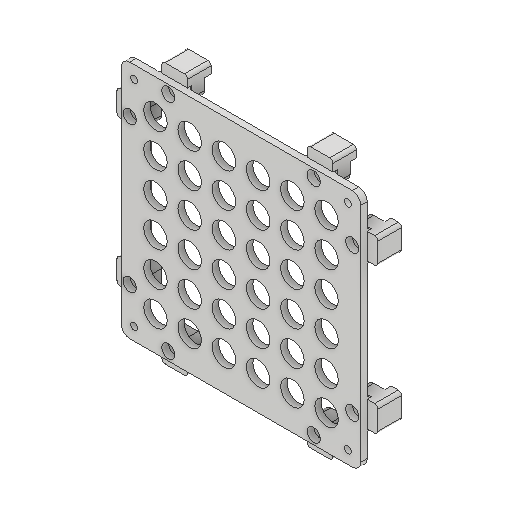
# Autodesk Inventor part: 3DP_PLA_Test_Tube_Plate
Saved by Autodesk Inventor 2025 (Build 290162010, 162A)
## iProperties
Created: 2018-06-16
Part Number: 3DP_PLA_Test_Tube_Plate
Material: ABS Plastic
Document SubType Name: Modeling
Designer: Andrzej
Density: 1.06 g/cm^3
Appearance: Smooth - White
Author: Andrzej
Autodesk Inventor part; units mm, degrees
ref_plane "YZ Plane" through (0, 0, 0) normal (1, 0, 0) x (0, 1, 0)
ref_plane "XZ Plane" through (0, 0, 0) normal (0, 1, 0) x (-1, 0, 0)
ref_plane "XY Plane" through (0, 0, 0) normal (0, 0, 1) x (1, 0, 0)
sketch "Sketch1" plane through (0, 0, 0) normal (0, 0, 1) x (1, 0, 0)
  line L0 (-56, 56) -> (56, 56)
  line L1 (56, 56) -> (56, -56)
  line L2 (56, -56) -> (-56, -56)
  line L3 (-56, -56) -> (-56, 56)
  circle A0 centre (-40, 40) radius 5.5
  circle A1 centre (-24, 40) radius 5.5
  circle A2 centre (-8, 40) radius 5.5
  circle A3 centre (8, 40) radius 5.5
  circle A4 centre (24, 40) radius 5.5
  circle A5 centre (40, 40) radius 5.5
  circle A6 centre (-40, 24) radius 5.5
  circle A7 centre (-24, 24) radius 5.5
  circle A8 centre (-8, 24) radius 5.5
  circle A9 centre (8, 24) radius 5.5
  circle A10 centre (24, 24) radius 5.5
  circle A11 centre (40, 24) radius 5.5
  circle A12 centre (-40, 8) radius 5.5
  circle A13 centre (-24, 8) radius 5.5
  circle A14 centre (-8, 8) radius 5.5
  circle A15 centre (8, 8) radius 5.5
  circle A16 centre (24, 8) radius 5.5
  circle A17 centre (40, 8) radius 5.5
  circle A18 centre (-40, -8) radius 5.5
  circle A19 centre (-24, -8) radius 5.5
  circle A20 centre (-8, -8) radius 5.5
  circle A21 centre (8, -8) radius 5.5
  circle A22 centre (24, -8) radius 5.5
  circle A23 centre (40, -8) radius 5.5
  circle A24 centre (-40, -24) radius 5.5
  circle A25 centre (-24, -24) radius 5.5
  circle A26 centre (-8, -24) radius 5.5
  circle A27 centre (8, -24) radius 5.5
  circle A28 centre (24, -24) radius 5.5
  circle A29 centre (40, -24) radius 5.5
  circle A30 centre (-40, -40) radius 5.5
  circle A31 centre (-24, -40) radius 5.5
  circle A32 centre (-8, -40) radius 5.5
  circle A33 centre (8, -40) radius 5.5
  circle A34 centre (24, -40) radius 5.5
  circle A35 centre (40, -40) radius 5.5
  point P0 (0, 0)
  point P1 (-50, 50)
  point P2 (50, 50)
  point P3 (-50, -50)
  point P4 (50, -50)
  dimension "d0" = 112
  dimension "d1" = 112
  dimension "d2" = 11
  dimension "d3" = 16
  dimension "d4" = 16
  dimension "d7" = 16
  dimension "d10" = 16
  dimension "d19" = 6
  dimension "d20" = 6
  dimension "d23" = 6
  dimension "d25" = 6
  dimension "d34" = 56
  dimension "d35" = 56
  constraints: 36 centre point, 8 end point, 2 horizontal, 2 horizontal alignment, 2 parallel, 2 vertical alignment, 1 perpendicular, 1 vertical, 70 other
  measures "d0" distance of L1.end L2.end
  measures "d1" distance of L0.end L1.end
  measures "d2" diameter of A0
  measures "d3" distance from line of L3 A0.centre
  measures "d4" distance from line of L0 A0.centre
  measures "d7" distance of A0.centre A1.centre
  measures "d10" distance of A0.centre A6.centre
  measures "d19" distance from line of L3 point (-50, 50)
  measures "d20" distance from line of L0 point (-50, 50)
  measures "d23" distance from line of L2 point (-50, -50)
  measures "d25" distance from line of L1 point (50, 50)
  measures "d34" distance from line of point (0, 0) L2
  measures "d35" distance from line of point (0, 0) L3
extrude "Extrusion2" add sketch "Sketch1" along normal blind 3
hole "Hole1" at (50, 50, 0) at (-50, -50, 0) at (-50, 50, 0) at (50, -50, 0) direction (0, 0, 1) diameter 3.25 end through all
fillet "Fillet1" radius 4 4 edges at (56, 56, 1.5) (56, -56, 1.5) (-56, -56, 1.5) (-56, 56, 1.5)
sketch "Sketch3" plane through (0, 0, 0) normal (0, 0, -1) x (-1, 0, 0)
  arc A0 (56, 52) -> (52, 56) centre (52, 52) ccw projected
  line L0 (52, 56) -> (-52, 56) projected
  arc A1 (-52, 56) -> (-56, 52) centre (-52, 52) ccw projected
  line L1 (-56, 52) -> (-56, -52) projected
  arc A2 (-56, -52) -> (-52, -56) centre (-52, -52) ccw projected
  line L2 (-52, -56) -> (52, -56) projected
  arc A3 (52, -56) -> (56, -52) centre (52, -52) ccw projected
  line L3 (56, -52) -> (56, 52) projected
  circle A4 centre (50, 50) radius 1.625 projected
  circle A5 centre (-50, 50) radius 1.625 projected
  circle A6 centre (50, -50) radius 1.625 projected
  circle A7 centre (-40, -40) radius 5.5 projected
  circle A8 centre (-24, -40) radius 5.5 projected
  circle A9 centre (-8, -40) radius 5.5 projected
  circle A10 centre (8, -40) radius 5.5 projected
  circle A11 centre (24, -40) radius 5.5 projected
  circle A12 centre (40, -40) radius 5.5 projected
  circle A13 centre (-40, -24) radius 5.5 projected
  circle A14 centre (-24, -24) radius 5.5 projected
  circle A15 centre (-8, -24) radius 5.5 projected
  circle A16 centre (8, -24) radius 5.5 projected
  circle A17 centre (24, -24) radius 5.5 projected
  circle A18 centre (40, -24) radius 5.5 projected
  circle A19 centre (-40, -8) radius 5.5 projected
  circle A20 centre (-24, -8) radius 5.5 projected
  circle A21 centre (-8, -8) radius 5.5 projected
  circle A22 centre (8, -8) radius 5.5 projected
  circle A23 centre (24, -8) radius 5.5 projected
  circle A24 centre (40, -8) radius 5.5 projected
  circle A25 centre (-40, 8) radius 5.5 projected
  circle A26 centre (-24, 8) radius 5.5 projected
  circle A27 centre (-8, 8) radius 5.5 projected
  circle A28 centre (8, 8) radius 5.5 projected
  circle A29 centre (24, 8) radius 5.5 projected
  circle A30 centre (40, 8) radius 5.5 projected
  circle A31 centre (-40, 24) radius 5.5 projected
  circle A32 centre (-24, 24) radius 5.5 projected
  circle A33 centre (-8, 24) radius 5.5 projected
  circle A34 centre (8, 24) radius 5.5 projected
  circle A35 centre (24, 24) radius 5.5 projected
  circle A36 centre (40, 24) radius 5.5 projected
  circle A37 centre (-40, 40) radius 5.5 projected
  circle A38 centre (-24, 40) radius 5.5 projected
  circle A39 centre (-8, 40) radius 5.5 projected
  circle A40 centre (8, 40) radius 5.5 projected
  circle A41 centre (24, 40) radius 5.5 projected
  circle A42 centre (40, 40) radius 5.5 projected
  circle A43 centre (-50, -50) radius 1.625 projected
  line L4 (-52, -56) -> (52, -56) projected
  line L5 (40, -56) -> (28, -56)
  line L6 (28, -56) -> (28, -61)
  line L7 (28, -61) -> (40, -61)
  line L8 (40, -61) -> (40, -56)
  line L9 (40, -56) -> (28, -56)
  line L10 (28, -56) -> (28, -48)
  line L11 (28, -48) -> (40, -48)
  line L12 (40, -48) -> (40, -56)
  line L13 (0, 62.6646) -> (0, -67.1052)
  line L14 (75.0583, 0) -> (-85.8021, 0)
  line L15 (-40, -56) -> (-28, -56)
  line L16 (-28, -56) -> (-28, -61)
  line L17 (-28, -61) -> (-40, -61)
  line L18 (-40, -61) -> (-40, -56)
  line L19 (-40, -56) -> (-28, -56)
  line L20 (-28, -56) -> (-28, -48)
  line L21 (-28, -48) -> (-40, -48)
  line L22 (-40, -48) -> (-40, -56)
  line L23 (40, 56) -> (28, 56)
  line L24 (28, 56) -> (28, 61)
  line L25 (28, 61) -> (40, 61)
  line L26 (40, 61) -> (40, 56)
  line L27 (40, 56) -> (28, 56)
  line L28 (28, 56) -> (28, 48)
  line L29 (28, 48) -> (40, 48)
  line L30 (40, 48) -> (40, 56)
  line L31 (-28, 56) -> (-28, 48)
  line L32 (-28, 48) -> (-40, 48)
  line L33 (-40, 48) -> (-40, 56)
  line L34 (-40, 56) -> (-28, 56)
  line L35 (-40, 56) -> (-28, 56)
  line L36 (-28, 61) -> (-40, 61)
  line L37 (-40, 61) -> (-40, 56)
  line L38 (-28, 56) -> (-28, 61)
  line L39 (-48, -28) -> (-48, -40)
  line L40 (-48, -40) -> (-56, -40)
  line L41 (-56, -28) -> (-48, -28)
  line L42 (-56, -40) -> (-56, -28)
  line L43 (-56, -40) -> (-56, -28)
  line L44 (-61, -40) -> (-56, -40)
  line L45 (-61, -28) -> (-61, -40)
  line L46 (-56, -28) -> (-61, -28)
  line L47 (-48, 28) -> (-48, 40)
  line L48 (-56, 28) -> (-48, 28)
  line L49 (-48, 40) -> (-56, 40)
  line L50 (-56, 40) -> (-56, 28)
  line L51 (-56, 40) -> (-56, 28)
  line L52 (-56, 28) -> (-61, 28)
  line L53 (-61, 28) -> (-61, 40)
  line L54 (-61, 40) -> (-56, 40)
  line L55 (56, -28) -> (48, -28)
  line L56 (48, -28) -> (48, -40)
  line L57 (56, -28) -> (61, -28)
  line L58 (48, -40) -> (56, -40)
  line L59 (56, -40) -> (56, -28)
  line L60 (56, -40) -> (56, -28)
  line L61 (61, -28) -> (61, -40)
  line L62 (61, -40) -> (56, -40)
  line L63 (48, 40) -> (56, 40)
  line L64 (61, 28) -> (61, 40)
  line L65 (56, 28) -> (61, 28)
  line L66 (61, 40) -> (56, 40)
  line L67 (48, 28) -> (48, 40)
  line L68 (56, 28) -> (48, 28)
  line L69 (56, 40) -> (56, 28)
  line L70 (56, 40) -> (56, 28)
  point P0 (0, 0)
  point P1 (56, 28)
  point P2 (-28, 56)
  point P3 (-56, 28)
  point P4 (-56, -28)
  point P5 (-28, -56)
  point P6 (56, 28)
  point P7 (-28, 56)
  point P8 (-56, 28)
  point P9 (-56, -28)
  point P10 (-28, -56)
  dimension "d36" = 12
  dimension "d37" = 5
  dimension "d38" = 8
  dimension "d39" = 16
  dimension "d42" = 270
  constraints: 132 end point, 21 symmetric about line, 11 point on line, 4 parallel, 3 horizontal, 2 perpendicular, 1 vertical, 61 other
  measures "d36" distance of L7.end L6.end
  measures "d37" distance of L6.end L5.end
  measures "d38" distance of L9.end L10.end
  measures "d39" distance between parallel lines of L3 L8
extrude "Extrusion3" add sketch "Sketch3" along normal blind 8 contours L3 L68 L67 L63 | L30 L29 L28 L0 | L3 L58 L56 L55 | L31 L32 L33 L0 | L2 L22 L21 L20 | L10 L11 L12 L2 | L1 L49 L47 L48 | L41 L39 L40 L1
extrude "Extrusion4" add sketch "Sketch3" along normal blind 11 contours L66 L64 L65 L3 | L0 L24 L25 L26 | L57 L61 L62 L3 | L0 L37 L36 L38 | L16 L17 L18 L2 | L2 L8 L7 L6 | L52 L53 L54 L1 | L1 L44 L45 L46
sketch "Sketch4" plane through (0, 0, -8) normal (0, 0, -1) x (-1, 0, 0)
  line L0 (28, -48) -> (28, -56) projected
  line L1 (40, -48) -> (28, -48) projected
  line L2 (48, -40) -> (56, -40) projected
  line L3 (48, -28) -> (48, -40) projected
  line L4 (48, 28) -> (56, 28) projected
  line L5 (48, 40) -> (48, 28) projected
  line L6 (40, 48) -> (40, 56) projected
  line L7 (28, 48) -> (40, 48) projected
  line L8 (-28, 48) -> (-28, 56) projected
  line L9 (-40, 48) -> (-28, 48) projected
  line L10 (-48, 40) -> (-56, 40) projected
  line L11 (-48, 28) -> (-48, 40) projected
  line L12 (-48, -28) -> (-56, -28) projected
  line L13 (-48, -40) -> (-48, -28) projected
  line L14 (-40, -48) -> (-40, -56) projected
  line L15 (-28, -48) -> (-40, -48) projected
  circle A0 centre (34, -52) radius 3.1
  line L16 (0, -63.7987) -> (0, 70.21)
  circle A1 centre (-34, -52) radius 3.1
  circle A2 centre (52, -34) radius 3.1
  circle A3 centre (52, 34) radius 3.1
  circle A4 centre (34, 52) radius 3.1
  circle A5 centre (-34, 52) radius 3.1
  circle A6 centre (-52, 34) radius 3.1
  circle A7 centre (-52, -34) radius 3.1
  line L17 (-40, -56) -> (-28, -56) projected
  line L18 (-28, -56) -> (-28, -48) projected
  line L19 (-56, -28) -> (-56, -40) projected
  line L20 (-56, -40) -> (-48, -40) projected
  line L21 (-56, 40) -> (-56, 28) projected
  line L22 (-56, 28) -> (-48, 28) projected
  line L23 (-28, 56) -> (-40, 56) projected
  line L24 (-40, 56) -> (-40, 48) projected
  line L25 (40, 56) -> (28, 56) projected
  line L26 (28, 56) -> (28, 48) projected
  line L27 (56, 28) -> (56, 40) projected
  line L28 (56, 40) -> (48, 40) projected
  line L29 (56, -40) -> (56, -28) projected
  line L30 (56, -28) -> (48, -28) projected
  line L31 (28, -56) -> (40, -56) projected
  line L32 (40, -56) -> (40, -48) projected
  point P0 (0, 0)
  point P1 (63.7987, 0)
  point P2 (0, 63.7987)
  point P3 (-63.7987, 0)
  dimension "d48" = 6.2
  dimension "d49" = 4
  dimension "d53" = 360
  constraints: 8 centre point, 2 end point, 1 symmetric about line, 1 vertical, 22 other
  measures "d48" diameter of A0
  measures "d49" distance from line of L1 A0.centre
extrude "Extrusion5" cut sketch "Sketch4" against normal blind 3.2 contours A0 | A1 | A2 | A3 | A4 | A5 | A6 | A7
fillet "Fillet2" radius 3 16 edges at (-48, -28, -4) (-48, -40, -4) (-40, -48, -4) (-28, -48, -4) (28, -48, -4) (40, -48, -4) (48, -40, -4) (48, -28, -4) (48, 40, -4) (48, 28, -4) (28, 48, -4) (40, 48, -4) (-40, 48, -4) (-28, 48, -4) (-48, 28, -4) (-48, 40, -4)
fillet "Fillet3" radius 2 40 edges at (28.8787, -48.8787, 0) (34, -48, 0) (39.1213, -48.8787, 0) (40, -53.5, 0) (28, -53.5, 0) (53.5, -28, 0) (48, -34, 0) (48.8787, -39.1213, 0) (53.5, -40, 0) (48.8787, -28.8787, 0) (48.8787, 28.8787, 0) (53.5, 28, 0) (48.8787, 39.1213, 0) (53.5, 40, 0) (48, 34, 0) (28.8787, 48.8787, 0) (34, 48, 0) (39.1213, 48.8787, 0) (40, 53.5, 0) (28, 53.5, 0) (-39.1213, 48.8787, 0) (-34, 48, 0) (-28.8787, 48.8787, 0) (-28, 53.5, 0) (-40, 53.5, 0) (-48.8787, 39.1213, 0) (-48, 34, 0) (-48.8787, 28.8787, 0) (-53.5, 28, 0) (-53.5, 40, 0) (-48.8787, -28.8787, 0) (-48, -34, 0) (-48.8787, -39.1213, 0) (-53.5, -40, 0) (-53.5, -28, 0) (-39.1213, -48.8787, 0) (-40, -53.5, 0) (-28.8787, -48.8787, 0) (-28, -53.5, 0) (-34, -48, 0)
sketch "Sketch5" plane through (0, 0, -11) normal (0, 0, -1) x (-1, 0, 0)
  circle A0 centre (50, 50) radius 1.625 projected
  circle A1 centre (-50, 50) radius 1.625 projected
  circle A2 centre (50, -50) radius 1.625 projected
  circle A3 centre (-50, -50) radius 1.625 projected
  circle A4 centre (-40, -40) radius 5.5 projected
  circle A5 centre (-24, -40) radius 5.5 projected
  circle A6 centre (-8, -40) radius 5.5 projected
  circle A7 centre (8, -40) radius 5.5 projected
  circle A8 centre (24, -40) radius 5.5 projected
  circle A9 centre (40, -40) radius 5.5 projected
  circle A10 centre (-40, -24) radius 5.5 projected
  circle A11 centre (-24, -24) radius 5.5 projected
  circle A12 centre (-8, -24) radius 5.5 projected
  circle A13 centre (8, -24) radius 5.5 projected
  circle A14 centre (24, -24) radius 5.5 projected
  circle A15 centre (40, -24) radius 5.5 projected
  circle A16 centre (-40, -8) radius 5.5 projected
  circle A17 centre (-24, -8) radius 5.5 projected
  circle A18 centre (-8, -8) radius 5.5 projected
  circle A19 centre (8, -8) radius 5.5 projected
  circle A20 centre (24, -8) radius 5.5 projected
  circle A21 centre (40, -8) radius 5.5 projected
  circle A22 centre (-40, 8) radius 5.5 projected
  circle A23 centre (-24, 8) radius 5.5 projected
  circle A24 centre (-8, 8) radius 5.5 projected
  circle A25 centre (8, 8) radius 5.5 projected
  circle A26 centre (24, 8) radius 5.5 projected
  circle A27 centre (40, 8) radius 5.5 projected
  circle A28 centre (-40, 24) radius 5.5 projected
  circle A29 centre (-24, 24) radius 5.5 projected
  circle A30 centre (-8, 24) radius 5.5 projected
  circle A31 centre (8, 24) radius 5.5 projected
  circle A32 centre (24, 24) radius 5.5 projected
  circle A33 centre (40, 24) radius 5.5 projected
  circle A34 centre (-40, 40) radius 5.5 projected
  circle A35 centre (-24, 40) radius 5.5 projected
  circle A36 centre (-8, 40) radius 5.5 projected
  circle A37 centre (8, 40) radius 5.5 projected
  circle A38 centre (24, 40) radius 5.5 projected
  circle A39 centre (40, 40) radius 5.5 projected
  arc A40 (56, 52) -> (52, 56) centre (52, 52) ccw projected
  line L0 (56, 52) -> (56, -52) projected
  arc A41 (52, -56) -> (56, -52) centre (52, -52) ccw projected
  line L1 (52, -56) -> (-52, -56) projected
  arc A42 (-56, -52) -> (-52, -56) centre (-52, -52) ccw projected
  line L2 (-56, -52) -> (-56, 52) projected
  arc A43 (-52, 56) -> (-56, 52) centre (-52, 52) ccw projected
  line L3 (-52, 56) -> (52, 56) projected
  arc A44 (56.2, 52) -> (52, 56.2) centre (52, 52) ccw
  line L4 (56.2, 52) -> (56.2, -52)
  arc A45 (52, -56.2) -> (56.2, -52) centre (52, -52) ccw
  line L5 (52, -56.2) -> (-52, -56.2)
  arc A46 (-56.2, -52) -> (-52, -56.2) centre (-52, -52) ccw
  line L6 (-56.2, -52) -> (-56.2, 52)
  arc A47 (-52, 56.2) -> (-56.2, 52) centre (-52, 52) ccw
  line L7 (-52, 56.2) -> (52, 56.2)
  point P0 (0, 0)
  dimension "d59" = 0.2
  constraints: 8 end point, 8 point on circle, 4 centre point, 7 other
  measures "d59" distance between parallel lines of L3 L7
extrude "Extrusion6" cut sketch "Sketch5" against normal up to surface (3 mm away) contours A0 | A1 | A2 | A3 | A4 | A5 | A6 | A7 | A8 | A9 | A10 | A11 | A12 | A13 | A14 | A15 | A16 | A17 | A18 | A19 | A20 | A21 | A22 | A23 | A24 | A25 | A26 | A27 | A28 | A29 | A30 | A31 | A32 | A33 | A34 | A35 | A36 | A37 | A38 | A39 | L0 A41 L1 A42 L2 A43 L3 A40 | L4 A45 L5 A46 L6 A47 L7 A44
fillet "Fillet4" radius 1.5 16 edges at (-28, -61, -5.5) (-40, -61, -5.5) (-61, -40, -5.5) (-61, -28, -5.5) (-61, 28, -5.5) (-61, 40, -5.5) (-40, 61, -5.5) (-28, 61, -5.5) (28, 61, -5.5) (40, 61, -5.5) (61, 40, -5.5) (61, 28, -5.5) (61, -28, -5.5) (61, -40, -5.5) (40, -61, -5.5) (28, -61, -5.5)
sketch "Sketch6" plane through (0, 0, 0) normal (0, 0, -1) x (-1, 0, 0)
  line L0 (51, 28) -> (61, 28) projected
  line L1 (56, -26) -> (56, 26) projected
  line L2 (56, 28) -> (56, 26) projected
  line L3 (56, -28) -> (56, -26) projected
  line L4 (51, -28) -> (61, -28) projected
  line L5 (53, 28) -> (53, -28)
  point P0 (0, 0)
  point P1 (56.2, 28)
  point P2 (56.2, -28)
  dimension "d63" = 3
  constraints: 2 end point, 2 point on line, 1 perpendicular
  measures "d63" distance between parallel lines of L1 L5
extrude "Extrusion7" add sketch "Sketch6" along normal up to surface (8 mm away)
sketch "Sketch7" plane through (0, 0, 3) normal (0, 0, 1) x (1, 0, 0)
  circle A0 centre (34, -52) radius 3.1 projected
  circle A1 centre (52, -34) radius 3.1 projected
  circle A2 centre (52, 34) radius 3.1 projected
  circle A3 centre (34, 52) radius 3.1 projected
  circle A4 centre (-34, 52) radius 3.1 projected
  circle A5 centre (-52, 34) radius 3.1 projected
  circle A6 centre (-52, -34) radius 3.1 projected
  circle A7 centre (-34, -52) radius 3.1 projected
  point P0 (0, 0)
extrude "Extrusion8" cut sketch "Sketch7" against normal blind 3.2
equation "\"d0\" = d1"
equation "\"d3\" = d4"
equation "\"d20\" = d19"
equation "\"d23\" = d19"
equation "\"d25\" = d19"
equation "\"d34\" = 0.5 * d1"
equation "\"d35\" = 0.5 * d0"
body "Solid2"
